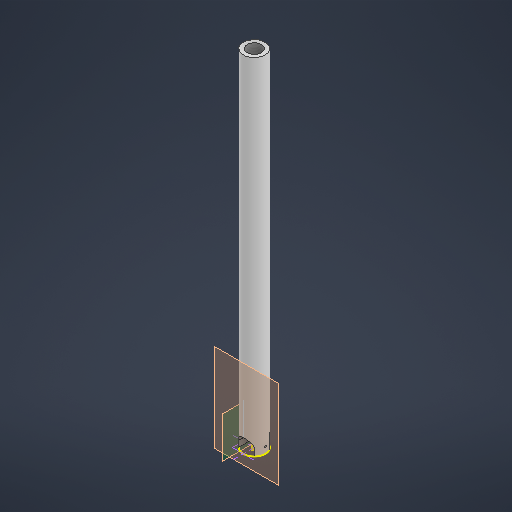
# Autodesk Inventor part: Output link body
Saved by Autodesk Inventor 2026.3 (Build 303398000, 398)
## iProperties
Created: 2026-07-24
Part Number: Output link body
Material: Generic
Document SubType Name: Sheet Metal
Designer: matot
Density: 1 g/cm^3
Sheet Metal Rule: Default_mm
Appearance: Default
Author: matot
Autodesk Inventor part; units mm, degrees
ref_plane "YZ Plane" through (0, 0, 0) normal (1, 0, 0) x (0, 1, 0)
ref_plane "XZ Plane" through (0, 0, 0) normal (0, 1, 0) x (-1, 0, 0)
ref_plane "XY Plane" through (0, 0, 0) normal (0, 0, 1) x (1, 0, 0)
sketch "Sketch1" plane through (0, 0, 0) normal (0, 1, 0) x (-1, 0, 0)
  circle A0 centre (0, 0) radius 17.5
  dimension "d0" = 35
  constraints: 1 centre point, 1 coincident
  measures "d0" diameter of A0
extrude "Extrusion1" add sketch "Sketch1" along normal blind 550
sketch "Sketch2" plane through (0, 550, 0) normal (0, 1, 0) x (1, 0, 0)
  circle A0 centre (0, 0) radius 22.5
  dimension "d3" = 45
  constraints: 2 coincident, 1 centre point
  measures "d3" diameter of A0
hole "Hole1" at (0, 550, 0) direction (0, -1, 0) diameter 22.8349 depth 40 tip angle 118 thread size "M25x2" class "6H" standard "ISO Metric profile"
sketch "Sketch3" plane through (0, 0, 0) normal (0, -1, 0) x (1, 0, 0)
  circle A0 centre (0, 0) radius 17.5 projected
  point P0 (0, 17.5)
  constraints: 1 vertical alignment, 1 other
ref_plane "Work Plane1" through (0, 0, 17.5) normal (0, 0, 1) x (1, 0, 0)
sketch "Sketch4" plane through (0, 0, 17.5) normal (0, 0, 1) x (1, 0, 0)
  line L0 (17.5, 0) -> (-17.5, 0) projected
  arc A0 (12.5, 10) -> (-12.5, 10) centre (0, 10) ccw
  line L1 (-12.5, 10) -> (-12.5, 0)
  line L2 (12.5, 10) -> (12.5, 0)
  point P0 (0, 0)
  dimension "d11" = 10
  dimension "d12" = 25
  constraints: 4 end point, 2 perpendicular, 2 point on circle, 2 point on line, 2 tangent, 1 centre point, 1 coincident
  measures "d11" distance from line of L0 point (0, 10)
  measures "d12" diameter of A0
extrude "Extrusion2" cut sketch "Sketch4" against normal through all
sketch "Sketch5" plane through (0, 0, 0) normal (0, -1, 0) x (1, 0, 0)
  arc A0 (-12.5, 12.2474) -> (-12.5, -12.2474) centre (0, 0) ccw projected
  point P0 (-17.5, 0)
  constraints: 1 point on circle
ref_plane "Work Plane2" through (-17.5, 0, 0) normal (-1, 0, 0) x (0, -1, 0)
sketch "Sketch6" plane through (-17.5, 0, 0) normal (-1, 0, 0) x (0, -1, 0)
  line L0 (0, 12.2474) -> (0, -12.2474) projected
  point P0 (0, 0)
  point P1 (-10, 0)
  point P2 (0, 0)
  dimension "d15" = 10
  constraints: 1 midpoint
  measures "d15" distance of point (0, 0) point (-10, 0)
hole "Hole2" at (-17.5, 10, 0) direction (1, 0, 0) diameter 3.242 end through all thread size "M4x0.7" class "6H" standard "ISO Metric profile"
equation "\"BendRadius\" = Thickness"
equation "\"BendReliefWidth\" = Thickness"
equation "\"BendReliefDepth\" = 0.5 * Thickness"
equation "\"CornerReliefSize\" = 4 * Thickness"
equation "\"MinimumRemnant\" = 2 * Thickness"
equation "\"TransitionRadius\" = BendRadius"
equation "\"JacobiRadiusSize\" = BendRadius"
equation "\"GapSize\" = Thickness"
equation "\"Thickness\" = 0.5"
body "Solid1"
